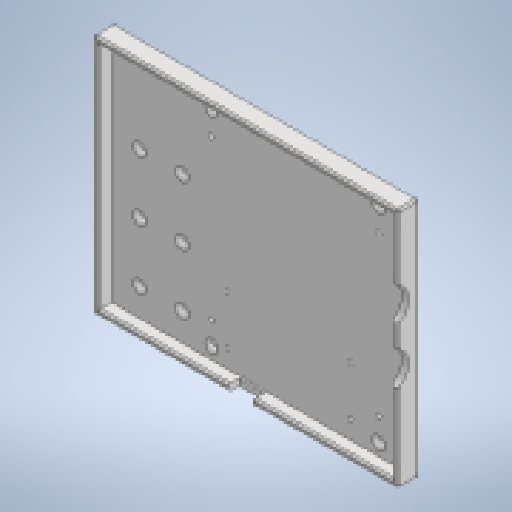
# Autodesk Inventor part: support
Saved by Autodesk Inventor 2024 (Build 280153000, 153)
## iProperties
Created: 2024-03-12
Part Number: support
Material: Générique
Document SubType Name: Modeling
Designer: phaly
Density: 1 g/cm^3
Appearance: Par défaut
Author: phaly
Autodesk Inventor part; units mm, degrees
ref_plane "YZ Plane" through (0, 0, 0) normal (1, 0, 0) x (0, 1, 0)
ref_plane "XZ Plane" through (0, 0, 0) normal (0, 1, 0) x (-1, 0, 0)
ref_plane "XY Plane" through (0, 0, 0) normal (0, 0, 1) x (1, 0, 0)
sketch "Esquisse1" plane through (0, 0, 0) normal (0, 0, 1) x (1, 0, 0)
  line L0 (0, 114) -> (144, 114)
  line L1 (144, 114) -> (144, 0)
  line L2 (144, 0) -> (0, 0)
  line L3 (0, 0) -> (0, 114)
  line L4 (3, 111) -> (141, 111)
  line L5 (141, 111) -> (141, 3)
  line L6 (141, 3) -> (3, 3)
  line L7 (3, 3) -> (3, 111)
  line L8 (0, -22.8) -> (0, 136.8) projected
  line L9 (-28.8, 0) -> (172.8, 0) projected
  point P0 (0, 0)
  dimension "d0" = 114
  dimension "d1" = 144
  dimension "d2" = 3
  dimension "d3" = 3
  dimension "d4" = 3
  dimension "d5" = 3
  constraints: 16 end point, 4 parallel, 2 collinear, 2 horizontal, 2 perpendicular
  measures "d0" distance of L2.end L0.start
  measures "d1" distance of L0.start L0.end
  measures "d2" distance between parallel lines of L0 L4
  measures "d3" distance between parallel lines of L2 L6
  measures "d4" distance between parallel lines of L3 L7
  measures "d5" distance between parallel lines of L1 L5
extrude "Extrusion1" add sketch "Esquisse1" along normal blind 10
sketch "Esquisse2" plane through (0, 0, 0) normal (0, 0, -1) x (-1, 0, 0)
  line L0 (0, 114) -> (-144, 114)
  line L1 (-144, 114) -> (-144, 0)
  line L2 (-144, 0) -> (0, 0)
  line L3 (0, 0) -> (0, 114)
  line L4 (0, 114) -> (0, 0) projected
  line L5 (-144, 114) -> (0, 114) projected
  line L6 (0, 0) -> (-144, 0) projected
  line L7 (-144, 0) -> (-144, 114) projected
  constraints: 8 end point, 4 collinear, 2 parallel, 1 horizontal, 1 perpendicular
extrude "Extrusion2" add sketch "Esquisse2" against normal blind 4
sketch "Esquisse7" plane through (0, 0, 0) normal (0, 0, -1) x (-1, 0, 0)
  arc A0 (-119, 10) -> (-117, 8) centre (-117, 10) ccw projected
  line L0 (-119, 10) -> (-119, 36) projected
  arc A1 (-117, 38) -> (-119, 36) centre (-117, 36) ccw projected
  line L1 (-117, 38) -> (-56, 38) projected
  arc A2 (-54, 36) -> (-56, 38) centre (-56, 36) ccw projected
  line L2 (-54, 36) -> (-54, 10) projected
  arc A3 (-56, 8) -> (-54, 10) centre (-56, 10) ccw projected
  line L3 (-56, 8) -> (-117, 8) projected
  line L4 (-111, 9) -> (-61, 9) projected
  line L5 (-61, 9) -> (-61, 14) projected
  line L6 (-61, 14) -> (-111, 14) projected
  line L7 (-111, 14) -> (-111, 9) projected
  circle A4 centre (-115.5, 34.5) radius 1.75 projected
  circle A5 centre (-57.5, 34.5) radius 1.75 projected
  circle A6 centre (-57.5, 11.5) radius 1.75 projected
  circle A7 centre (-115.5, 11.5) radius 1.75 projected
  circle A8 centre (-36, 72) radius 1 projected
  circle A9 centre (-36, 44) radius 1 projected
  line L8 (-44, 8) -> (-26.5, 8) projected
  line L9 (-44, 80) -> (-44, 8) projected
  line L10 (-26.5, 80) -> (-44, 80) projected
  line L11 (-26.5, 8) -> (-26.5, 80) projected
  circle A10 centre (-16, 44) radius 1 projected
  circle A11 centre (-16, 16) radius 1 projected
  line L12 (-25, 8) -> (-8, 8) projected
  line L13 (-25, 80) -> (-25, 8) projected
  line L14 (-8, 80) -> (-25, 80) projected
  line L15 (-8, 8) -> (-8, 80) projected
  circle A12 centre (-16, 72) radius 1 projected
  circle A13 centre (-36, 16) radius 1 projected
  point P0 (0, 0)
  point P1 (-16, 16)
  point P2 (-16, 44)
  point P3 (-36, 44)
  point P4 (-36, 72)
  point P5 (-36, 16)
  point P6 (-16, 72)
  dimension "d105" = 28
  dimension "d106" = 28
  dimension "d107" = 20
  dimension "d108" = 20
  dimension "d109" = 20
  dimension "d110" = 28
  constraints: 8 coincident
  measures "d105" distance of point (-36, 16) point (-36, 44)
  measures "d106" distance of point (-16, 16) point (-16, 44)
  measures "d107" distance of point (-16, 44) point (-36, 44)
  measures "d108" distance of point (-16, 16) point (-36, 16)
  measures "d109" distance of point (-16, 72) point (-36, 72)
  measures "d110" distance of point (-16, 44) point (-16, 72)
hole "Perçage1" at (57.5, 11.5, 0) at (57.5, 34.5, 0) at (115.5, 11.5, 0) at (115.5, 34.5, 0) at (16, 44, 0) at (36, 44, 0) at (36, 72, 0) at (16, 16, 0) at (36, 16, 0) at (16, 72, 0) direction (0, 0, 1) diameter 2.5 end through all
sketch "Esquisse8" plane through (0, 0, 0) normal (0, -1, 0) x (1, 0, 0)
  line L0 (66.5, 8) -> (73.5, 8) projected
  line L1 (73.5, 8) -> (73.5, 12) projected
  line L2 (66.5, 12) -> (73.5, 12) projected
  line L3 (66.5, 8) -> (66.5, 12) projected
  line L4 (76, 5) -> (64, 5)
  line L5 (64, 5) -> (64, 10)
  line L6 (64, 10) -> (76, 10)
  line L7 (76, 10) -> (76, 5)
  line L8 (0, 10) -> (144, 10) projected
  line L9 (70, -1.8749) -> (70, 11.0144)
  point P0 (0, 0)
  dimension "d43" = 12
  dimension "d44" = 3.5
  dimension "d45" = 5
  constraints: 10 end point, 2 parallel, 1 collinear, 1 horizontal, 1 perpendicular, 1 vertical, 1 other
  measures "d43" distance of L4.start L4.end
  measures "d44" distance between parallel lines of L1 L9
  measures "d45" distance of L6.end L4.start
extrude "Extrusion6" cut sketch "Esquisse8" against normal blind 10 contours L3 L6 L9 L0 | L0 L9 L4 L5 L6 L3 | L9 L6 L1 L0 | L0 L1 L6 L7 L4 L9
sketch "Esquisse11" plane through (0, 0, 0) normal (0, 0, -1) x (-1, 0, 0)
  line L0 (0, 0) -> (-144, 0) projected
  line L1 (-144, 114) -> (0, 114) projected
  line L2 (-144, 0) -> (-144, 114) projected
  point P0 (-50, 105.5)
  point P1 (-129, 105.5)
  point P2 (-129, 8.5)
  point P3 (-50, 8.5)
  point P4 (-50, 94.5)
  point P5 (-50, 19.5)
  point P6 (-129, 19.5)
  point P7 (-129, 94.5)
  dimension "d54" = 79
  dimension "d55" = 79
  dimension "d56" = 97
  dimension "d57" = 97
  dimension "d58" = 8.5
  dimension "d59" = 8.5
  dimension "d60" = 8.5
  dimension "d68" = 15
  dimension "d69" = 79
  dimension "d70" = 79
  dimension "d71" = 75
  dimension "d72" = 75
  dimension "d73" = 11
  dimension "d74" = 11
  dimension "d75" = 15
  dimension "d76" = 19.5
  measures "d54" distance of point (-129, 105.5) point (-50, 105.5)
  measures "d55" distance of point (-129, 8.5) point (-50, 8.5)
  measures "d56" distance of point (-50, 8.5) point (-50, 105.5)
  measures "d57" distance of point (-129, 8.5) point (-129, 105.5)
  measures "d58" distance from line of L0 point (-50, 8.5)
  measures "d59" distance from line of L0 point (-129, 8.5)
  measures "d60" distance from line of L1 point (-50, 105.5)
  measures "d68" distance from line of L2 point (-129, 8.5)
  measures "d69" distance of point (-129, 94.5) point (-50, 94.5)
  measures "d70" distance of point (-129, 19.5) point (-50, 19.5)
  measures "d71" distance of point (-129, 19.5) point (-129, 94.5)
  measures "d72" distance of point (-50, 19.5) point (-50, 94.5)
  measures "d73" distance of point (-50, 8.5) point (-50, 19.5)
  measures "d74" distance of point (-129, 8.5) point (-129, 19.5)
  measures "d75" distance from line of L2 point (-129, 19.5)
  measures "d76" distance from line of L1 point (-50, 94.5)
hole "Perçage2" at (50, 105.5, 0) at (129, 105.5, 0) at (129, 8.5, 0) at (50, 8.5, 0) at (50, 94.5, 0) at (50, 19.5, 0) at (129, 94.5, 0) at (129, 19.5, 0) direction (0, 0, 1) diameter 2.5 end through all
sketch "Esquisse12" plane through (144, 0, 0) normal (1, 0, 0) x (0, 0, -1)
  circle A0 centre (-14, 49.2786) radius 8 projected
  circle A1 centre (-14, 75.2786) radius 8 projected
  arc A2 (-10, 41.2164) -> (-10, 57.3409) centre (-14, 49.2786) ccw
  arc A3 (-10, 67.2164) -> (-10, 83.3409) centre (-14, 75.2786) ccw
  line L0 (-10, 41.2164) -> (-10, 57.3409)
  line L1 (-10, 67.2164) -> (-10, 83.3409)
  line L2 (-10, 0) -> (-10, 114) projected
  point P0 (0, 0)
  dimension "d77" = 9
  dimension "d78" = 9
  constraints: 4 end point, 4 point on circle, 3 collinear, 2 centre point, 2 coincident, 1 vertical
  measures "d77" radius of A2
  measures "d78" radius of A3
extrude "Extrusion8" cut sketch "Esquisse12" against normal up to surface (3 mm away) contours A0 L0 | A0 L0 A2 | A1 L1 | A1 L1 A3 picked at (-9.549, 47.2969) picked at (-9.549, 73.2969)
sketch "Esquisse13" plane through (141, 3, 4) normal (-1, 0, 0) x (0, 0, 1)
  line L0 (0.5, 56.2409) -> (0.5, 62.2409)
  line L1 (5, 62.2409) -> (5, 56.2409)
  arc A0 (5, 62.2409) -> (0.5, 62.2409) centre (2.75, 62.2409) ccw
  arc A1 (0.5, 56.2409) -> (5, 56.2409) centre (2.75, 56.2409) ccw
  line L2 (6, 64.2164) -> (6, 54.3409) projected
  point P0 (-4, -3)
  dimension "d82" = 4.5
  dimension "d84" = 6
  dimension "d87" = 1.9
  dimension "d88" = 1
  constraints: 4 end point, 4 point on circle, 4 tangent, 2 centre point, 1 parallel
  measures "d82" distance between parallel lines of L0 L1
  measures "d84" distance of A1.centre A0.centre
  measures "d87" vertical distance of L2.end A1.centre
  measures "d88" distance between parallel lines of L1 L2
extrude "Extrusion9" cut sketch "Esquisse13" against normal blind 1.5
sketch "Esquisse14" plane through (0, 0, 0) normal (0, 0, -1) x (-1, 0, 0)
  circle A0 centre (-138.5, 87.2786) radius 1 projected
  circle A1 centre (-138.5, 37.2786) radius 1 projected
  point P0 (0, 0)
  point P1 (-138.5, 87.2786)
  constraints: 2 coincident
hole "Perçage3" at (138.5, 87.2786, 0) at (138.5, 37.2786, 0) direction (0, 0, 1) diameter 2 depth 8 tip angle 118
fillet "Congé2" radius 1 22 edges at (110, 0, 10) (144, 20.6082, 10) (141, 22.1082, 10) (108.5, 3, 10) (144, 62.2786, 10) (141, 62.2786, 10) (144, 98.6704, 10) (141, 97.1704, 10) (72, 111, 10) (72, 114, 10) (0, 57, 10) (3, 57, 10) (0, 57, 0) (0, 114, 5) (72, 114, 0) (144, 114, 5) (144, 0, 5) (144, 57, 0) (72, 0, 0) (32, 0, 10) (33.5, 3, 10) (0, 0, 5)
fillet "Congé3" radius 2 10 edges at (129, 93.25, 0) (129, 18.25, 0) (50, 18.25, 0) (50, 93.25, 0) (57.5, 33.25, 0) (115.5, 33.25, 0) (115.5, 10.25, 0) (57.5, 10.25, 0) (138.5, 36.2786, 0) (138.5, 86.2786, 0)
fillet "Congé4" radius 2 10 edges at (129, 7.25, 4) (129, 104.25, 4) (50, 104.25, 4) (36, 70.75, 4) (36, 42.75, 4) (16, 42.75, 4) (16, 14.75, 4) (50, 7.25, 4) (36, 14.75, 4) (16, 70.75, 4)
equation "\"d3\" = d2"
equation "\"d4\" = d3"
equation "\"d5\" = d4"
equation "\"d55\" = d54"
equation "\"d57\" = d56"
equation "\"d59\" = d58"
equation "\"d60\" = d58"
equation "\"d69\" = d54"
equation "\"d70\" = d55"
equation "\"d72\" = d71"
equation "\"d74\" = d73"
equation "\"d75\" = d68"
equation "\"d78\" = d77"
